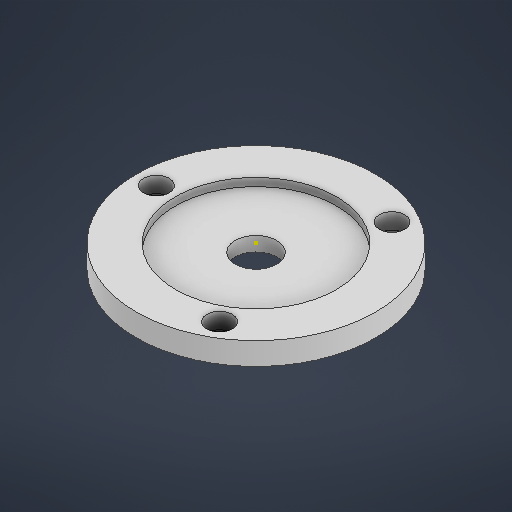
# Autodesk Inventor part: 1.1.5.UpperSta.Plate
Saved by Autodesk Inventor 2026.1 (Build 301233020, 233B)
## iProperties
Created: 2025-10-08
Part Number: 1.1.5.UpperSta.Plate
Material: Genérico
Document SubType Name: Modeling
Designer: vitos
Density: 1 g/cm^3
Appearance: Valor por defecto
Author: vitos
Autodesk Inventor part; units mm, degrees
ref_plane "YZ Plane" through (0, 0, 0) normal (1, 0, 0) x (0, 1, 0)
ref_plane "XZ Plane" through (0, 0, 0) normal (0, 1, 0) x (-1, 0, 0)
ref_plane "XY Plane" through (0, 0, 0) normal (0, 0, 1) x (1, 0, 0)
sketch "Boceto1" plane through (0, 0, 0) normal (0, 1, 0) x (-1, 0, 0)
  circle A0 centre (0, 0) radius 75
  circle A1 centre (62.5, 0) radius 5
  circle A2 centre (62.5, 0) radius 8
  circle A3 centre (0, 0) radius 13
  circle A4 centre (-31.25, -54.1266) radius 5
  circle A5 centre (-31.25, -54.1266) radius 8
  circle A6 centre (-31.25, 54.1266) radius 5
  circle A7 centre (-31.25, 54.1266) radius 8
  dimension "d0" = 150
  dimension "d1" = 10
  dimension "d2" = 16
  dimension "d3" = 26
  dimension "d4" = 10
  dimension "d5" = 16
  dimension "d6" = 10
  dimension "d7" = 16
  constraints: 8 centre point, 5 coincident
  measures "d0" diameter of A0
  measures "d1" diameter of A1
  measures "d2" diameter of A2
  measures "d3" diameter of A3
  measures "d4" diameter of A4
  measures "d5" diameter of A5
  measures "d6" diameter of A6
  measures "d7" diameter of A7
extrude "Extrusión1" add sketch "Boceto1" along normal blind 14 contours A0 | A2 | A5 | A7
sketch "Boceto2" plane through (0, 14, 0) normal (0, 1, 0) x (1, 0, 0)
  point P0 (0, 0)
sketch "Boceto3" plane through (0, 14, 0) normal (0, 1, 0) x (1, 0, 0)
  circle A0 centre (0, 0) radius 50.5
  circle A1 centre (-62.5, 0) radius 8
  circle A2 centre (31.25, 54.1266) radius 5 projected
  circle A3 centre (31.25, 54.1266) radius 8
  circle A4 centre (31.25, -54.1266) radius 5 projected
  circle A5 centre (31.25, -54.1266) radius 8
  dimension "d10" = 101
  dimension "d11" = 16
  dimension "d12" = 16
  dimension "d13" = 16
  constraints: 4 centre point, 3 coincident
  measures "d10" diameter of A0
  measures "d11" diameter of A1
  measures "d12" diameter of A3
  measures "d13" diameter of A5
extrude "Extrusión2" cut sketch "Boceto3" against normal blind 10 contours A1 | A2 | A3 | A4 | A5
extrude "Extrusión3" cut sketch "Boceto3" against normal blind 5 contours A0
